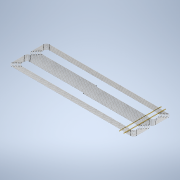
# Autodesk Inventor part: coil7conductors
Saved by Autodesk Inventor 2021 (Build 250183000, 183)
## iProperties
Created: 2022-01-18
Part Number: coil7conductors
Material: Generic
Document SubType Name: Modeling
Designer: avan411
Density: 1 g/cm^3
Appearance: Default
Author: avan411
Autodesk Inventor part; units mm, degrees
ref_plane "XZ Plane" through (0, 0, 0) normal (0, 1, 0) x (-1, 0, 0)
ref_plane "XY Plane" through (0, 0, 0) normal (0, 0, 1) x (1, 0, 0)
sketch "Sketch1" plane through (0, 0, 0) normal (0, 1, 0) x (-1, 0, 0)
  line L0 (0, 0) -> (-500, 0) construction
  line L1 (-500, 0) -> (-500, -150) construction
  line L2 (-500, -150) -> (500, -150) construction
  line L3 (500, -150) -> (500, -7.35) construction
  line L4 (500, -7.35) -> (-493.7, -7.35) construction
  line L5 (-493.7, -7.35) -> (-493.7, -144.0107) construction
  line L6 (-493.7, -144.0107) -> (493.7, -144.0107) construction
  line L7 (493.7, -144.0107) -> (493.7, -14.7) construction
  line L8 (493.7, -14.7) -> (-487.4, -14.7) construction
  line L9 (-487.4, -14.7) -> (-487.4, -138.0214) construction
  line L10 (-487.4, -138.0214) -> (487.4, -138.0214) construction
  line L11 (487.4, -138.0214) -> (487.4, -22.05) construction
  line L12 (487.4, -22.05) -> (0, -22.05) construction
  line L13 (0, 0) -> (0, -7.35) construction
  line L14 (0, -7.35) -> (0, -14.7) construction
  line L15 (0, -14.7) -> (0, -22.05) construction
  line L16 (0, -138.0214) -> (0, -144.0107) construction
  line L17 (0, -144.0107) -> (0, -150) construction
  line L18 (0, 0) -> (500, 0)
  line L19 (500, 0) -> (500, 150) construction
  line L20 (500, 150) -> (-500, 150) construction
  line L21 (-500, 150) -> (-500, 7.35) construction
  line L22 (-500, 7.35) -> (493.7, 7.35) construction
  line L23 (493.7, 7.35) -> (493.7, 143.7) construction
  line L24 (493.7, 143.7) -> (-493.7, 143.7) construction
  line L25 (-493.7, 143.7) -> (-493.7, 14.7) construction
  line L26 (-493.7, 14.7) -> (487.4, 14.7) construction
  line L27 (487.4, 14.7) -> (487.4, 137.4) construction
  line L28 (487.4, 137.4) -> (-487.4, 137.4) construction
  line L29 (-487.4, 137.4) -> (-487.4, 22.05) construction
  line L30 (0, 0) -> (0, 7.35) construction
  line L31 (0, 7.35) -> (0, 14.7) construction
  line L32 (0, 137.4) -> (0, 143.7) construction
  line L33 (0, 143.7) -> (0, 150) construction
  arc A0 (487.4, -46.05) -> (463.4, -22.05) centre (463.4, -46.05) ccw
  arc A1 (493.7, -38.7) -> (469.7, -14.7) centre (469.7, -38.7) ccw
  arc A2 (500, -31.35) -> (476, -7.35) centre (476, -31.35) ccw
  arc A3 (463.4, -138.0214) -> (487.4, -114.0214) centre (463.4, -114.0214) ccw
  arc A4 (469.7, -144.0107) -> (493.7, -120.0107) centre (469.7, -120.0107) ccw
  arc A5 (476, -150) -> (500, -126) centre (476, -126) ccw
  arc A6 (-463.4, -14.7) -> (-487.4, -38.7) centre (-463.4, -38.7) ccw
  arc A7 (-493.7, 38.7) -> (-469.7, 14.7) centre (-469.7, 38.7) ccw
  arc A8 (-500, 31.35) -> (-476, 7.35) centre (-476, 31.35) ccw
  arc A9 (-500, -126) -> (-476, -150) centre (-476, -126) ccw
  arc A10 (-493.7, -120.0107) -> (-469.7, -144.0107) centre (-469.7, -120.0107) ccw
  arc A11 (-487.4, -114.0214) -> (-463.4, -138.0214) centre (-463.4, -114.0214) ccw
  arc A12 (-476, 150) -> (-500, 126) centre (-476, 126) ccw
  arc A13 (-469.7, 143.7) -> (-493.7, 119.7) centre (-469.7, 119.7) ccw
  arc A14 (463.4, 14.7) -> (487.4, 38.7) centre (463.4, 38.7) ccw
  arc A15 (469.7, 7.35) -> (493.7, 31.35) centre (469.7, 31.35) ccw
  arc A16 (476, 0) -> (500, 24) centre (476, 24) ccw
  arc A17 (487.4, 113.4) -> (463.4, 137.4) centre (463.4, 113.4) ccw
  arc A18 (-469.7, -7.35) -> (-493.7, -31.35) centre (-469.7, -31.35) ccw
  arc A19 (-476, 0) -> (-500, -24) centre (-476, -24) ccw
  arc A20 (-463.4, 137.4) -> (-487.4, 113.4) centre (-463.4, 113.4) ccw
  arc A21 (500, 126) -> (476, 150) centre (476, 126) ccw
  arc A22 (493.7, 119.7) -> (469.7, 143.7) centre (469.7, 119.7) ccw
  line L34 (463.4, -138.0214) -> (-463.4, -138.0214)
  line L35 (-463.4, -14.7) -> (469.7, -14.7)
  line L36 (469.7, -144.0107) -> (-469.7, -144.0107)
  line L37 (476, -150) -> (-476, -150)
  line L38 (-469.7, -7.35) -> (476, -7.35)
  line L39 (-476, 0) -> (476, 0)
  line L40 (500, -31.35) -> (500, -126)
  line L41 (493.7, -38.7) -> (493.7, -120.0107)
  line L42 (487.4, -114.0214) -> (487.4, -46.05)
  line L43 (-487.4, -38.7) -> (-487.4, -114.0214)
  line L44 (-493.7, -120.0107) -> (-493.7, -31.35)
  line L45 (-500, -24) -> (-500, -126)
  line L46 (-500, 31.35) -> (-500, 126)
  line L47 (-493.7, 119.7) -> (-493.7, 38.7)
  line L48 (500, 24) -> (500, 126)
  line L49 (493.7, 119.7) -> (493.7, 31.35)
  line L50 (487.4, 113.4) -> (487.4, 38.7)
  line L51 (469.7, 7.35) -> (-476, 7.35)
  line L52 (-469.7, 14.7) -> (463.4, 14.7)
  line L53 (463.4, 137.4) -> (-463.4, 137.4)
  line L54 (-469.7, 143.7) -> (469.7, 143.7)
  line L55 (476, 150) -> (-476, 150)
  line L56 (-487.4, 113.4) -> (-487.4, 46.05)
  line L57 (463.4, -22.05) -> (-457.1, -22.05)
  line L58 (0, -22.05) -> (-481.1, -22.05) construction
  line L59 (-481.1, -22.05) -> (-481.1, -132.0321) construction
  line L60 (-481.1, -132.0321) -> (481.1, -132.0321) construction
  line L61 (481.1, -132.0321) -> (481.1, -29.4) construction
  line L62 (481.1, -29.4) -> (-474.8, -29.4) construction
  line L63 (-474.8, -126.0428) -> (474.8, -126.0428) construction
  line L64 (474.8, -126.0428) -> (474.8, -36.75) construction
  line L65 (474.8, -36.75) -> (-468.5, -36.75) construction
  line L66 (-468.5, -120.0535) -> (468.5, -120.0535) construction
  line L67 (468.5, -120.0535) -> (468.5, -44.1) construction
  line L68 (468.5, -44.1) -> (-462.2, -44.1) construction
  line L69 (-462.2, -114.0642) -> (462.2, -114.0642) construction
  line L70 (462.2, -114.0642) -> (462.2, -51.45) construction
  line L71 (462.2, -51.45) -> (0, -51.45) construction
  line L72 (0, -22.05) -> (0, -29.4) construction
  line L73 (0, -29.4) -> (0, -36.75) construction
  line L74 (0, -36.75) -> (0, -44.1) construction
  line L75 (0, -44.1) -> (0, -51.45) construction
  line L76 (0, -138.0214) -> (0, -132.0321) construction
  line L77 (0, -132.0321) -> (0, -126.0428) construction
  line L78 (0, -126.0428) -> (0, -120.0535) construction
  line L79 (0, -120.0535) -> (0, -114.0642) construction
  line L80 (-500, -44.1) -> (-493.7, -44.1) construction
  line L81 (-493.7, -44.1) -> (-487.4, -44.1) construction
  line L82 (-487.4, -44.1) -> (-481.1, -44.1) construction
  line L83 (-462.2, -114.0642) -> (-462.2, -44.1) construction
  line L84 (-468.5, -120.0535) -> (-468.5, -36.75) construction
  line L85 (-468.5, -44.1) -> (-462.2, -44.1) construction
  line L86 (-474.8, -29.4) -> (-474.8, -126.0428) construction
  line L87 (-481.1, -44.1) -> (-474.8, -44.1) construction
  line L88 (-474.8, -44.1) -> (-468.5, -44.1) construction
  line L89 (500, -51.45) -> (493.7, -51.45) construction
  line L90 (493.7, -51.45) -> (487.4, -51.45) construction
  line L91 (474.8, -51.45) -> (468.5, -51.45) construction
  line L92 (468.5, -51.45) -> (462.2, -51.45) construction
  line L93 (487.4, -51.45) -> (481.1, -51.45) construction
  line L94 (481.1, -51.45) -> (474.8, -51.45) construction
  arc A23 (-457.1, -22.05) -> (-481.1, -46.05) centre (-457.1, -46.05) ccw
  line L95 (-481.1, -46.05) -> (-481.1, -108.0321)
  arc A24 (-481.1, -108.0321) -> (-457.1, -132.0321) centre (-457.1, -108.0321) ccw
  line L96 (-457.1, -132.0321) -> (457.1, -132.0321)
  arc A25 (457.1, -132.0321) -> (481.1, -108.0321) centre (457.1, -108.0321) ccw
  line L97 (481.1, -108.0321) -> (481.1, -53.4)
  arc A26 (481.1, -53.4) -> (457.1, -29.4) centre (457.1, -53.4) ccw
  line L98 (457.1, -29.4) -> (-450.8, -29.4)
  arc A27 (-450.8, -29.4) -> (-474.8, -53.4) centre (-450.8, -53.4) ccw
  line L99 (-474.8, -53.4) -> (-474.8, -102.0428)
  arc A28 (-474.8, -102.0428) -> (-450.8, -126.0428) centre (-450.8, -102.0428) ccw
  line L100 (-450.8, -126.0428) -> (450.8, -126.0428)
  arc A29 (450.8, -126.0428) -> (474.8, -102.0428) centre (450.8, -102.0428) ccw
  line L101 (474.8, -102.0428) -> (474.8, -60.75)
  arc A30 (474.8, -60.75) -> (450.8, -36.75) centre (450.8, -60.75) ccw
  line L102 (450.8, -36.75) -> (-444.5, -36.75)
  arc A31 (-444.5, -36.75) -> (-468.5, -60.75) centre (-444.5, -60.75) ccw
  line L103 (-468.5, -60.75) -> (-468.5, -96.0535)
  arc A32 (-468.5, -96.0535) -> (-444.5, -120.0535) centre (-444.5, -96.0535) ccw
  line L104 (-444.5, -120.0535) -> (444.5, -120.0535)
  arc A33 (444.5, -120.0535) -> (468.5, -96.0535) centre (444.5, -96.0535) ccw
  line L105 (468.5, -96.0535) -> (468.5, -68.1)
  arc A34 (468.5, -68.1) -> (444.5, -44.1) centre (444.5, -68.1) ccw
  line L106 (444.5, -44.1) -> (-438.2, -44.1)
  arc A35 (-438.2, -44.1) -> (-462.2, -68.1) centre (-438.2, -68.1) ccw
  line L107 (-462.2, -68.1) -> (-462.2, -90.0642)
  arc A36 (-462.2, -90.0642) -> (-438.2, -114.0642) centre (-438.2, -90.0642) ccw
  line L108 (-438.2, -114.0642) -> (438.2, -114.0642)
  arc A37 (438.2, -114.0642) -> (462.2, -90.0642) centre (438.2, -90.0642) ccw
  line L109 (462.2, -90.0642) -> (462.2, -75.45)
  arc A38 (462.2, -75.45) -> (438.2, -51.45) centre (438.2, -75.45) ccw
  line L110 (438.2, -51.45) -> (0, -51.45)
  line L111 (-487.4, 22.05) -> (481.1, 22.05) construction
  line L112 (481.1, 22.05) -> (481.1, 131.1) construction
  line L113 (481.1, 131.1) -> (-481.1, 131.1) construction
  line L114 (-481.1, 131.1) -> (-481.1, 29.4) construction
  line L115 (-481.1, 29.4) -> (474.8, 29.4) construction
  line L116 (474.8, 29.4) -> (474.8, 124.8) construction
  line L117 (474.8, 124.8) -> (-474.8, 124.8) construction
  line L118 (-474.8, 124.8) -> (-474.8, 36.75) construction
  line L119 (-474.8, 36.75) -> (468.5, 36.75) construction
  line L120 (468.5, 36.75) -> (468.5, 118.5) construction
  line L121 (468.5, 118.5) -> (-468.5, 118.5) construction
  line L122 (-468.5, 118.5) -> (-468.5, 44.1) construction
  line L123 (-468.5, 44.1) -> (462.2, 44.1) construction
  line L124 (462.2, 44.1) -> (462.2, 112.2) construction
  line L125 (462.2, 112.2) -> (-462.2, 112.2) construction
  line L126 (-462.2, 112.2) -> (-462.2, 51.45) construction
  line L127 (-462.2, 51.45) -> (0, 51.45) construction
  line L128 (0, 137.4) -> (0, 131.1) construction
  line L129 (0, 131.1) -> (0, 124.8) construction
  line L130 (0, 124.8) -> (0, 118.5) construction
  line L131 (0, 118.5) -> (0, 112.2) construction
  line L132 (-500, 51.45) -> (-493.7, 51.45) construction
  line L133 (-493.7, 51.45) -> (-487.4, 51.45) construction
  line L134 (-487.4, 51.45) -> (-481.1, 51.45) construction
  line L135 (-481.1, 51.45) -> (-474.8, 51.45) construction
  line L136 (-474.8, 51.45) -> (-468.5, 51.45) construction
  line L137 (-468.5, 51.45) -> (-462.2, 51.45) construction
  line L138 (500, 44.1) -> (493.7, 44.1) construction
  line L139 (487.4, 44.1) -> (493.7, 44.1) construction
  line L140 (487.4, 44.1) -> (481.1, 44.1) construction
  line L141 (481.1, 44.1) -> (474.8, 44.1) construction
  line L142 (474.8, 44.1) -> (468.5, 44.1) construction
  line L143 (468.5, 44.1) -> (462.2, 44.1) construction
  line L144 (0, 29.4) -> (0, 36.75) construction
  line L145 (0, 36.75) -> (0, 44.1) construction
  line L146 (0, 44.1) -> (0, 51.45) construction
  line L147 (0, 22.05) -> (0, 14.7) construction
  line L148 (0, 22.05) -> (0, 29.4) construction
  arc A39 (-487.4, 46.05) -> (-463.4, 22.05) centre (-463.4, 46.05) ccw
  line L149 (-463.4, 22.05) -> (457.1, 22.05)
  arc A40 (457.1, 22.05) -> (481.1, 46.05) centre (457.1, 46.05) ccw
  line L150 (481.1, 46.05) -> (481.1, 107.1)
  arc A41 (481.1, 107.1) -> (457.1, 131.1) centre (457.1, 107.1) ccw
  line L151 (457.1, 131.1) -> (-457.1, 131.1)
  arc A42 (-457.1, 131.1) -> (-481.1, 107.1) centre (-457.1, 107.1) ccw
  line L152 (-481.1, 107.1) -> (-481.1, 53.4)
  arc A43 (-481.1, 53.4) -> (-457.1, 29.4) centre (-457.1, 53.4) ccw
  line L153 (-457.1, 29.4) -> (450.8, 29.4)
  arc A44 (450.8, 29.4) -> (474.8, 53.4) centre (450.8, 53.4) ccw
  line L154 (474.8, 53.4) -> (474.8, 100.8)
  arc A45 (474.8, 100.8) -> (450.8, 124.8) centre (450.8, 100.8) ccw
  line L155 (450.8, 124.8) -> (-450.8, 124.8)
  arc A46 (-450.8, 124.8) -> (-474.8, 100.8) centre (-450.8, 100.8) ccw
  line L156 (-474.8, 100.8) -> (-474.8, 60.75)
  arc A47 (-474.8, 60.75) -> (-450.8, 36.75) centre (-450.8, 60.75) ccw
  line L157 (-450.8, 36.75) -> (444.5, 36.75)
  arc A48 (444.5, 36.75) -> (468.5, 60.75) centre (444.5, 60.75) ccw
  line L158 (468.5, 60.75) -> (468.5, 94.5)
  arc A49 (468.5, 94.5) -> (444.5, 118.5) centre (444.5, 94.5) ccw
  line L159 (444.5, 118.5) -> (-444.5, 118.5)
  arc A50 (-444.5, 118.5) -> (-468.5, 94.5) centre (-444.5, 94.5) ccw
  line L160 (-468.5, 94.5) -> (-468.5, 68.1)
  arc A51 (-468.5, 68.1) -> (-444.5, 44.1) centre (-444.5, 68.1) ccw
  line L161 (-444.5, 44.1) -> (438.2, 44.1)
  arc A52 (438.2, 44.1) -> (462.2, 68.1) centre (438.2, 68.1) ccw
  line L162 (462.2, 68.1) -> (462.2, 88.2)
  arc A53 (462.2, 88.2) -> (438.2, 112.2) centre (438.2, 88.2) ccw
  line L163 (438.2, 112.2) -> (-438.2, 112.2)
  arc A54 (-438.2, 112.2) -> (-462.2, 88.2) centre (-438.2, 88.2) ccw
  line L164 (-462.2, 88.2) -> (-462.2, 75.45)
  arc A55 (-462.2, 75.45) -> (-438.2, 51.45) centre (-438.2, 75.45) ccw
  line L165 (-438.2, 51.45) -> (0, 51.45)
  dimension "d5" = 1000
  dimension "d6" = 150
  dimension "d11" = 12.6
  dimension "d13" = 150
  dimension "d16" = 12.6
  dimension "d18" = 0
  dimension "d19" = 24
  dimension "d100" = 44.1
  dimension "d102" = 35.9358
  dimension "d104" = 37.8
  dimension "d105" = 500
  dimension "d106" = 500
  constraints: 333 end point, 170 point on line, 117 tangent, 112 point on circle, 65 perpendicular, 56 centre point, 55 equal radius, 45 equal length, 25 collinear, 14 midpoint, 13 parallel, 6 horizontal, 4 vertical
  measures "d5" distance of L1.end L2.end
  measures "d6" distance of L0.end L1.end
  measures "d11" distance between parallel lines of L1 L9
  measures "d13" distance of L19.start L19.end
  measures "d16" distance between parallel lines of L20 L28
  measures "d18" distance from line of L13 L0.start
  measures "d19" radius of A11
  measures "d100" distance of L13.end L71.end
  measures "d102" distance of L79.end L17.end
  measures "d104" distance between parallel lines of L124 L48
  measures "d105" distance from line of L21 L0.start
  measures "d106" distance from line of L19 L0.start
sketch "Sketch2" plane through (0, 0, 0) normal (1, 0, 0) x (0, 1, 0)
  circle A0 centre (0, -51.45) radius 2.15
  point P0 (0, 0)
  point P1 (0, 51.45)
  dimension "d103" = 4.3
  constraints: 2 coincident, 1 centre point
  measures "d103" diameter of A0
ref_plane "Work Plane1" through (438.2, 0, 0) normal (1, 0, 0) x (0, 1, 0)
ref_plane "Work Plane2" through (404.5, 0, 0) normal (1, 0, 0) x (0, 1, 0)
sweep "Sweep4" add profiles "Sketch2" path "Sketch1" path curves L110 A38 L109 A37 L108 A36 L107 A35 L106 A34 L105 A33 L104 A32 L103 A31 L102 A30 L101 A29 L100 A28 L99 A27 L98 A26 L97 A25 L96 A24 L95 A23 L57 A0 L42 A3 L34 A11 L43 A6 L35 A1 L41 A4 L36 A10 L44 A18 L38 A2 L40 A5 L37 A9 L45 A19 L39 A16 L48 A21 L55 A12 L46 A8 L51 A15 L49 A22 L54 A13 L47 A7 L52 A14 L50 A17 L53 A20 L56 A39 L149 A40 L150 A41 L151 A42 L152 A43 L153 A44 L154 A45 L155 A46 L156 A47 L157 A48 L158 A49 L159 A50 L160 A51 L161 A52 L162 A53 L163 A54 L164 A55 L165
split body "Split3" result two bodies by plane through (404.5, 0, 0) normal (1, 0, 0) first body at (462.0757, -0.0664, 66.0795) (417.8333, 1.6446, 43.9672) (419.9333, 1.6286, 36.4853) (482.0912, 1.3191, 89.2) (488.3912, 1.3191, 90.95) (494.6912, 1.3191, 92.7) (500.9912, 1.3191, 94.45) (500.1328, 1.6446, -92) (494.6912, 1.3191, -60.9036) (487.2672, 1.6446, -88.9143) (480.8353, 1.6286, -87.3714) (475.7912, 1.3191, -69.6143) (417.8333, 1.6286, -37.0147) (451.0243, 0.0664, -45.8876)
split "Split4" plane through (438.2, 0, 0) removes the side toward (-1, 0, 0) bodies 2
move or copy body "Move Body2" bodies to move or copy 2 copy no translate (0, -4.3, 0)
loft "Loft17" add bodies 3 section 1 edges at (404.5, -2.15, 150) section 2 edges at (438.2, -6.45, 150)
loft "Loft18" add bodies 3 section 1 edges at (404.5, -2.15, 143.7) section 2 edges at (438.2, -6.45, 143.7)
loft "Loft19" add bodies 3 section 1 edges at (404.5, -2.15, 137.4) section 2 edges at (438.2, -6.45, 137.4)
loft "Loft20" add bodies 3 section 1 edges at (404.5, -2.15, 131.1) section 2 edges at (438.2, -6.45, 131.1)
loft "Loft21" add bodies 3 section 1 edges at (404.5, -2.15, 124.8) section 2 edges at (438.2, -6.45, 124.8)
loft "Loft22" add bodies 3 section 1 edges at (404.5, -2.15, 118.5) section 2 edges at (438.2, -6.45, 118.5)
loft "Loft23" add bodies 3 section 1 edges at (404.5, -2.15, 112.2) section 2 edges at (438.2, -6.45, 112.2)
loft "Loft24" add bodies 3 section 1 edges at (404.5, -2.15, 51.45) section 2 edges at (438.2, -6.45, 51.45)
loft "Loft25" add bodies 3 section 1 edges at (404.5, -2.15, 44.1) section 2 edges at (438.2, -6.45, 44.1)
loft "Loft26" add bodies 3 section 1 edges at (404.5, -2.15, 36.75) section 2 edges at (438.2, -6.45, 36.75)
loft "Loft27" add bodies 3 section 1 edges at (404.5, -2.15, 29.4) section 2 edges at (438.2, -6.45, 29.4)
loft "Loft28" add bodies 3 section 1 edges at (404.5, -2.15, 22.05) section 2 edges at (438.2, -6.45, 22.05)
loft "Loft29" add bodies 3 section 1 edges at (404.5, -2.15, 14.7) section 2 edges at (438.2, -6.45, 14.7)
loft "Loft30" add bodies 3 section 1 edges at (404.5, -2.15, 7.35) section 2 edges at (438.2, -6.45, 7.35)
loft "Loft31" add bodies 3 section 1 edges at (404.5, -2.15, 0) section 2 edges at (438.2, -6.45, 0)
loft "Loft32" add bodies 3 section 1 edges at (404.5, -2.15, -7.35) section 2 edges at (438.2, -6.45, -7.35)
loft "Loft33" add bodies 3 section 1 edges at (404.5, -2.15, -14.7) section 2 edges at (438.2, -6.45, -14.7)
loft "Loft34" add bodies 3 section 1 edges at (404.5, -2.15, -22.05) section 2 edges at (438.2, -6.45, -22.05)
loft "Loft35" add bodies 3 section 1 edges at (404.5, -2.15, -29.4) section 2 edges at (438.2, -6.45, -29.4)
loft "Loft36" add bodies 3 section 1 edges at (404.5, -2.15, -36.75) section 2 edges at (438.2, -6.45, -36.75)
loft "Loft37" add bodies 3 section 1 edges at (404.5, -2.15, -44.1) section 2 edges at (438.2, -6.45, -44.1)
loft "Loft38" add bodies 3 section 1 edges at (404.5, -2.15, -114.0642) section 2 edges at (438.2, -6.45, -114.0642)
loft "Loft39" add bodies 3 section 1 edges at (404.5, -2.15, -120.0535) section 2 edges at (438.2, -6.45, -120.0535)
loft "Loft40" add bodies 3 section 1 edges at (404.5, -2.15, -126.0428) section 2 edges at (438.2, -6.45, -126.0428)
loft "Loft41" add bodies 3 section 1 edges at (404.5, -2.15, -132.0321) section 2 edges at (438.2, -6.45, -132.0321)
loft "Loft42" add bodies 3 section 1 edges at (404.5, -2.15, -138.0214) section 2 edges at (438.2, -6.45, -138.0214)
loft "Loft43" add bodies 3 section 1 edges at (404.5, -2.15, -144.0107) section 2 edges at (438.2, -6.45, -144.0107)
loft "Loft44" add bodies 3 section 1 edges at (404.5, -2.15, -150) section 2 edges at (438.2, -6.45, -150)
body "Solid7"
body "Solid8"
